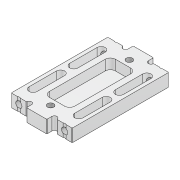
# Autodesk Inventor part: 16_010_FEMUR_BRIDGE_R1
Saved by Autodesk Inventor 2021.2 (Build 252289000, 289)
## iProperties
Created: 2020-07-26
Part Number: 16_010_FEMUR_BRIDGE_R1
Material: Aluminum 6061
Document SubType Name: Modeling
Designer: y6tada
Density: 2.7 g/cm^3
Appearance: Aluminum - Flat
Author: y6tada
Autodesk Inventor part; units mm, degrees
ref_plane "YZ Plane" through (0, 0, 0) normal (1, 0, 0) x (0, 1, 0)
ref_plane "XZ Plane" through (0, 0, 0) normal (0, 1, 0) x (-1, 0, 0)
ref_plane "XY Plane" through (0, 0, 0) normal (0, 0, 1) x (1, 0, 0)
sketch "Sketch1" plane through (0, 0, 0) normal (0, 1, 0) x (-1, 0, 0)
  line L0 (12, 19) -> (-12, 19)
  line L1 (-12, 19) -> (-12, -19)
  line L2 (-12, -19) -> (12, -19)
  line L3 (12, -19) -> (12, 19)
  line L4 (12, 19) -> (-12, -19) construction
  line L5 (-12, 19) -> (12, -19) construction
  point P0 (0, 0)
  dimension "d1" = 38
  dimension "d2" = 24
  constraints: 12 end point, 2 midpoint, 2 parallel, 1 horizontal, 1 perpendicular
  measures "d1" distance between parallel lines of L0 L2
  measures "d2" distance between parallel lines of L1 L3
extrude "Extrusion1" add sketch "Sketch1" along normal mid plane 5
sketch "Sketch2" plane through (0, 0, 0) normal (0, 1, 0) x (-1, 0, 0)
  line L0 (4, 21) -> (-4, 21)
  line L1 (-4, 21) -> (-4, -21)
  line L2 (-4, -21) -> (4, -21)
  line L3 (4, -21) -> (4, 21)
  line L4 (4, 21) -> (-4, -21) construction
  line L5 (-4, 21) -> (4, -21) construction
  line L6 (12, 19) -> (-12, 19) construction
  point P0 (0, 0)
  dimension "d5" = 2
  dimension "d6" = 8
  constraints: 12 end point, 2 midpoint, 2 parallel, 1 horizontal, 1 perpendicular
  measures "d5" distance between parallel lines of L0 L6
  measures "d6" distance of L0.start L0.end
extrude "Extrusion2" add sketch "Sketch2" along normal mid plane 5
sketch "Sketch3" plane through (0, 0, 0) normal (0, 1, 0) x (-1, 0, 0)
  line L0 (9, 19.8) -> (-9, 19.8) construction
  line L1 (-9, 19.8) -> (-9, -19.8) construction
  line L2 (-9, -19.8) -> (9, -19.8) construction
  line L3 (9, -19.8) -> (9, 19.8) construction
  line L4 (9, 19.8) -> (-9, -19.8) construction
  line L5 (-9, 19.8) -> (9, -19.8) construction
  line L6 (-4, 19) -> (-12, 19) construction
  line L7 (5, -19) -> (-5, -19) construction
  line L8 (-5, -19) -> (-5, 19) construction
  line L9 (-5, 19) -> (5, 19) construction
  line L10 (5, 19) -> (5, -19) construction
  line L11 (5, -19) -> (-5, 19) construction
  line L12 (-5, -19) -> (5, 19) construction
  line L13 (-4, 21) -> (-4, 19) construction
  point P0 (0, 0)
  dimension "d9" = 18
  dimension "d10" = 0.8
  dimension "d18" = 1
  constraints: 24 end point, 8 coincident, 4 midpoint, 4 parallel, 2 horizontal, 2 perpendicular, 1 collinear
  measures "d9" distance of L0.start L0.end
  measures "d10" distance between parallel lines of L6 L0
  measures "d18" distance from line of point (-5, 19) L13
hole "Hole1" at (-9, 0, -19.8) at (9, 0, -19.8) at (-9, 0, 19.8) at (9, 0, 19.8) at (-5, 0, 19) at (5, 0, 19) at (5, 0, -19) at (-5, 0, -19) direction (0, -1, 0) diameter 2 end through all both
sketch "Sketch4" plane through (0, 2.5, 0) normal (0, 1, 0) x (1, 0, 0)
  arc A0 (9.6, -19) -> (8.4, -19) centre (9, -19.8) ccw construction
  line L0 (9, -2.6) -> (9, -13.4) construction
  line L1 (7.4, -2.6) -> (7.4, -13.4)
  line L2 (10.6, -13.4) -> (10.6, -2.6)
  arc A1 (10.6, -2.6) -> (7.4, -2.6) centre (9, -2.6) ccw
  arc A2 (7.4, -13.4) -> (10.6, -13.4) centre (9, -13.4) ccw
  line L3 (9, -13.4) -> (9, -19.8) construction
  line L4 (11.2053, -15) -> (6.997, -15) construction
  line L5 (9.6, -19) -> (12, -19) construction
  line L6 (0, 0) -> (0, -18.6494) construction
  line L7 (-7.4, -2.6) -> (-7.4, -13.4)
  line L8 (-10.6, -13.4) -> (-10.6, -2.6)
  arc A3 (-7.4, -2.6) -> (-10.6, -2.6) centre (-9, -2.6) ccw
  arc A4 (-10.6, -13.4) -> (-7.4, -13.4) centre (-9, -13.4) ccw
  line L9 (0, 0) -> (15.9534, 0) construction
  line L10 (-6, 15) -> (6, 15)
  line L11 (6, 15) -> (6, -15)
  line L12 (6, -15) -> (-6, -15)
  line L13 (-6, -15) -> (-6, 15)
  line L14 (-6, 15) -> (6, -15) construction
  line L15 (6, 15) -> (-6, -15) construction
  line L16 (12, -19) -> (12, 19) construction
  line L17 (15.1424, -1) -> (0.2359, -1) construction
  line L18 (9, 2.6) -> (9, 13.4) construction
  line L19 (7.4, 2.6) -> (7.4, 13.4)
  line L20 (10.6, 13.4) -> (10.6, 2.6)
  arc A5 (7.4, 2.6) -> (10.6, 2.6) centre (9, 2.6) ccw
  arc A6 (10.6, 13.4) -> (7.4, 13.4) centre (9, 13.4) ccw
  arc A7 (-10.6, 2.6) -> (-7.4, 2.6) centre (-9, 2.6) ccw
  line L21 (-10.6, 13.4) -> (-10.6, 2.6)
  line L22 (-7.4, 2.6) -> (-7.4, 13.4)
  arc A8 (-7.4, 13.4) -> (-10.6, 13.4) centre (-9, 13.4) ccw
  point P0 (9, -8)
  point P1 (9, 8)
  dimension "d19" = 4
  dimension "d22" = 3.2
  dimension "d23" = 6
  dimension "d24" = 2
  constraints: 46 end point, 19 symmetric about line, 16 point on circle, 8 centre point, 6 tangent, 3 horizontal, 3 midpoint, 3 parallel, 3 vertical, 1 collinear, 1 perpendicular, 6 other
  measures "d19" distance between parallel lines of L5 L4
  measures "d22" distance between parallel lines of L2 L1
  measures "d23" distance between parallel lines of L16 L11
  measures "d24" diameter of L17 L9
extrude "Extrusion3" cut sketch "Sketch4" against normal blind 4
offset faces "Size1" outward 1 faces at (-6, 1.1667, -5) (6, 1.1667, 5)
offset faces "Size2" outward 2 faces at (-1.6667, 1.1667, 15) (-1.6667, -0.1667, -15)
sketch "Sketch7" plane through (0, 2.5, 0) normal (0, 1, 0) x (1, 0, 0)
  line L0 (5, -13) -> (-5, -13) construction
  line L1 (-5, 13) -> (5, 13) construction
  line L2 (5, -15.5) -> (-5, -15.5) construction
  line L3 (-5, 15.5) -> (5, 15.5) construction
  line L4 (-12, -19) -> (-9.6, -19) projected
  point P0 (0, 0)
  point P1 (0, -15.5)
  point P2 (0, 15.5)
  dimension "d42" = 2.5
  dimension "d43" = 2.5
  dimension "d51" = 3.5
  constraints: 4 end point, 2 midpoint, 2 parallel
  measures "d42" distance between parallel lines of L0 L2
  measures "d43" distance between parallel lines of L1 L3
  measures "d51" distance between parallel lines of L2 L4
hole "Hole3" at (0, 2.5, 15.5) at (0, 2.5, -15.5) direction (0, -1, 0) diameter 2.459 end through all thread size "M3x0.5" class "6H" standard "ISO Metric profile"
fillet "Fillet1" radius 2 4 edges at (5, 0.5, 13) (-5, 0.5, 13) (-5, 0.5, -13) (5, 0.5, -13)
chamfer "Chamfer1" distance 0.2 angle 45 12 edges at (12, 0, -19) (4, 0, -21) (-4, 0, -21) (-12, 0, -19) (12, 0, 19) (4, 0, 21) (-4, 0, 21) (-12, 0, 19) (-6, 0, 19) (6, 0, 19) (-6, 0, -19) (6, 0, -19)
sketch "Sketch6" plane through (3.8, 2.5, -21) normal (0, 0, -1) x (-1, 0, 0)
  line L0 (-4.6, -5) -> (-5.8, -5) construction
  line L1 (-4.6, 0) -> (-4.6, -5) construction
  line L2 (-5.8, 0) -> (-4.6, 0) construction
  line L3 (-5.8, -5) -> (-5.8, 0) construction
  line L4 (12.2, 0) -> (13.4, 0) construction
  line L5 (12.2, -5) -> (12.2, 0) construction
  line L6 (13.4, -5) -> (12.2, -5) construction
  line L7 (13.4, 0) -> (13.4, -5) construction
  line L8 (12.2, 0) -> (13.4, -5) construction
  line L9 (-5.8, 0) -> (-4.6, -5) construction
  point P0 (3.8, -2.5)
  point P1 (-5.2, -2.5)
  point P2 (12.8, -2.5)
  constraints: 4 end point, 2 midpoint, 1 parallel
hole "Hole2" at (9, 0, -21) at (-9, 0, -21) direction (0, 0, 1) diameter 2.459 depth 8.8 tip angle 118 thread size "M3x0.5" class "6H" standard "ISO Metric profile"
mirror "Mirror1" about plane through (0, 0, 0) normal (0, 0, 1) of "Hole2"
sketch "Sketch8" plane through (0, 2.5, 0) normal (0, 1, 0) x (1, 0, 0)
  circle A0 centre (0, -15.5) radius 1.2295 projected
  circle A1 centre (0, 15.5) radius 1.2295 projected
  arc A2 (-7.4, -2.6) -> (-10.6, -2.6) centre (-9, -2.6) ccw projected
  line L0 (-7.4, -2.6) -> (-7.4, -13.4) projected
  arc A3 (-10.6, -13.4) -> (-7.4, -13.4) centre (-9, -13.4) ccw projected
  line L1 (-10.6, -13.4) -> (-10.6, -2.6) projected
  line L2 (-10.6, 2.6) -> (-10.6, 13.4) projected
  arc A4 (-7.4, 13.4) -> (-10.6, 13.4) centre (-9, 13.4) ccw projected
  line L3 (-7.4, 13.4) -> (-7.4, 2.6) projected
  arc A5 (-10.6, 2.6) -> (-7.4, 2.6) centre (-9, 2.6) ccw projected
  line L4 (5, 11) -> (5, -11) projected
  arc A6 (3, -13) -> (5, -11) centre (3, -11) ccw projected
  line L5 (3, -13) -> (-3, -13) projected
  arc A7 (-5, -11) -> (-3, -13) centre (-3, -11) ccw projected
  line L6 (-5, -11) -> (-5, 11) projected
  arc A8 (-3, 13) -> (-5, 11) centre (-3, 11) ccw projected
  line L7 (-3, 13) -> (3, 13) projected
  arc A9 (5, 11) -> (3, 13) centre (3, 11) ccw projected
  line L8 (10.6, -2.6) -> (10.6, -13.4) projected
  arc A10 (7.4, -13.4) -> (10.6, -13.4) centre (9, -13.4) ccw projected
  line L9 (7.4, -13.4) -> (7.4, -2.6) projected
  arc A11 (10.6, -2.6) -> (7.4, -2.6) centre (9, -2.6) ccw projected
  arc A12 (7.4, 2.6) -> (10.6, 2.6) centre (9, 2.6) ccw projected
  line L10 (7.4, 2.6) -> (7.4, 13.4) projected
  arc A13 (10.6, 13.4) -> (7.4, 13.4) centre (9, 13.4) ccw projected
  line L11 (10.6, 13.4) -> (10.6, 2.6) projected
  line L12 (5.98, 18.801) -> (6.2, 19) projected
  arc A14 (4, 19) -> (5.98, 18.801) centre (5, 19) ccw projected
  line L13 (4, 19) -> (4, 20.8) projected
  line L14 (3.8, 21) -> (4, 20.8) projected
  line L15 (3.8, 21) -> (-3.8, 21) projected
  line L16 (-4, 20.8) -> (-3.8, 21) projected
  line L17 (-4, 20.8) -> (-4, 19) projected
  arc A15 (-5.98, 18.801) -> (-4, 19) centre (-5, 19) ccw projected
  line L18 (-6.2, 19) -> (-5.98, 18.801) projected
  line L19 (-6.2, 19) -> (-8.4, 19) projected
  arc A16 (-9.6, 19) -> (-8.4, 19) centre (-9, 19.8) ccw projected
  line L20 (-9.6, 19) -> (-11.8, 19) projected
  line L21 (-12, 18.8) -> (-11.8, 19) projected
  line L22 (-12, 18.8) -> (-12, -18.8) projected
  line L23 (-11.8, -19) -> (-12, -18.8) projected
  line L24 (-11.8, -19) -> (-9.6, -19) projected
  arc A17 (-8.4, -19) -> (-9.6, -19) centre (-9, -19.8) ccw projected
  line L25 (-8.4, -19) -> (-6.2, -19) projected
  line L26 (-5.98, -18.801) -> (-6.2, -19) projected
  arc A18 (-4, -19) -> (-5.98, -18.801) centre (-5, -19) ccw projected
  line L27 (-4, -19) -> (-4, -20.8) projected
  line L28 (-3.8, -21) -> (-4, -20.8) projected
  line L29 (-3.8, -21) -> (3.8, -21) projected
  line L30 (4, -20.8) -> (3.8, -21) projected
  line L31 (4, -20.8) -> (4, -19) projected
  arc A19 (5.98, -18.801) -> (4, -19) centre (5, -19) ccw projected
  line L32 (6.2, -19) -> (5.98, -18.801) projected
  line L33 (6.2, -19) -> (8.4, -19) projected
  arc A20 (9.6, -19) -> (8.4, -19) centre (9, -19.8) ccw projected
  line L34 (9.6, -19) -> (11.8, -19) projected
  line L35 (12, -18.8) -> (11.8, -19) projected
  line L36 (12, -18.8) -> (12, 18.8) projected
  line L37 (11.8, 19) -> (12, 18.8) projected
  line L38 (11.8, 19) -> (9.6, 19) projected
  arc A21 (8.4, 19) -> (9.6, 19) centre (9, 19.8) ccw projected
  line L39 (8.4, 19) -> (6.2, 19) projected
  point P0 (0, 0)
body "Solid1"
